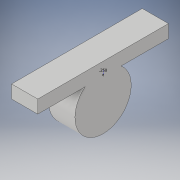
# Autodesk Inventor part: Part1
Saved by Autodesk Inventor 2019 (Build 230136000, 136)
## iProperties
Created: 2019-01-24
Part Number: Part1
Material: Generic
Document SubType Name: Modeling
Designer: pepin
Density: 1 g/cm^3
Appearance: Default
Author: pepin
Autodesk Inventor part; units mm, degrees
ref_plane "YZ Plane" through (0, 0, 0) normal (1, 0, 0) x (0, 1, 0)
ref_plane "XZ Plane" through (0, 0, 0) normal (0, 1, 0) x (-1, 0, 0)
ref_plane "XY Plane" through (0, 0, 0) normal (0, 0, 1) x (1, 0, 0)
sketch "Sketch1" plane through (0, 0, 0) normal (0, 0, 1) x (1, 0, 0)
  line L0 (0, 0) -> (-25.4, 0)
  line L1 (-25.4, 0) -> (-25.4, 12.7)
  line L2 (-25.4, 12.7) -> (0, 12.7)
  line L3 (0, 12.7) -> (0, 0)
  dimension "d0" = 25.4
  dimension "d1" = 12.7
  constraints: 8 end point, 2 parallel, 1 horizontal, 1 perpendicular
  measures "d0" distance of L1.end L2.end
  measures "d1" distance of L0.end L1.end
extrude "Extrusion1" add sketch "Sketch1" along normal mid plane 127
sketch "Sketch2" plane through (0, 0, 63.5) normal (1, 0, 0) x (0, 0, -1)
  line L0 (63.5, 0) -> (63.5, 6.35) construction
  dimension "d4" = 6.35
  constraints: 2 end point, 1 vertical
  measures "d4" distance of L0.start L0.end
sketch "Sketch3" plane through (0, 0, 63.5) normal (1, 0, 0) x (0, 0, -1)
  circle A0 centre (63.5, -20.9571) radius 27.3277
  point P0 (63.5, 0)
  constraints: 1 centre point
extrude "Extrusion2" add sketch "Sketch3" against normal blind 25.4
body "Solid1"
